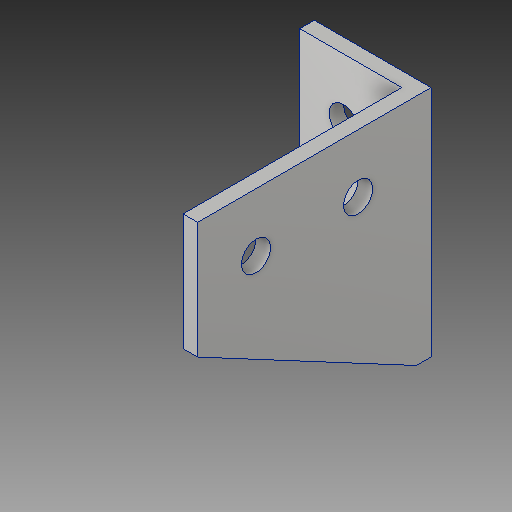
# Autodesk Inventor part: 15102898-16-P-0207
Saved by Autodesk Inventor 2017 (Build 210142000, 142)
## iProperties
Created: 2016-10-02
Part Number: 15102898-16-P-0207
Material: Aluminum 6061
Document SubType Name: Modeling
Designer: gus
Density: 2.7 g/cm^3
Appearance: Aluminum - Flat
Mass: 25.5302 g
Surface Area: 69.3547 cm^2
Volume: 9.45564 cm^3
Author: gus
Autodesk Inventor part; units mm, degrees
ref_plane "YZ Plane" through (0, 0, 0) normal (1, 0, 0) x (0, 1, 0)
ref_plane "XZ Plane" through (0, 0, 0) normal (0, 1, 0) x (-1, 0, 0)
ref_plane "XY Plane" through (0, 0, 0) normal (0, 0, 1) x (1, 0, 0)
sketch "Sketch1" plane through (0, 0, 0) normal (1, 0, 0) x (0, 1, 0)
  line L0 (-25.4, 0) -> (-50.8, -47.625)
  line L1 (-50.8, -47.625) -> (-50.8, -50.8)
  line L2 (-50.8, -50.8) -> (0, -50.8)
  line L3 (0, -50.8) -> (0, 0)
  line L4 (0, 0) -> (-25.4, 0)
  circle A0 centre (-12.7, -12.7) radius 3.175
  circle A1 centre (-12.7, -34.925) radius 3.175
  dimension "d1" = 3.175
  dimension "d2" = 50.8
  dimension "d3" = 50.8
  dimension "d4" = 25.4
  dimension "d5" = 6.35
  dimension "d6" = 6.35
  dimension "d7" = 15.875
  dimension "d8" = 12.7
  dimension "d9" = 12.7
  dimension "d10" = 12.7
  constraints: 10 end point, 3 perpendicular, 2 centre point, 1 coincident, 1 horizontal
  measures "d1" distance of L0.end L1.end
  measures "d2" distance of L1.end L2.end
  measures "d3" distance of L2.end L3.end
  measures "d4" distance of L3.end L0.start
  measures "d5" diameter of A0
  measures "d6" diameter of A1
  measures "d7" distance from line of L2 A1.centre
  measures "d8" distance from line of L3 A1.centre
  measures "d9" distance from line of L3 A0.centre
  measures "d10" distance from line of L4 A0.centre
extrude "Extrusion1" add sketch "Sketch1" along normal blind 3.175
sketch "Sketch2" plane through (0, 0, 0) normal (-1, 0, 0) x (0, 0, 1)
  line L0 (-50.8, -50.8) -> (-50.8, 0) projected
  line L1 (-50.8, 0) -> (0, 0) projected
  line L2 (-50.8, -50.8) -> (-47.625, -50.8)
  line L3 (-47.625, -50.8) -> (-47.625, 0)
  line L4 (-47.625, 0) -> (-50.8, 0)
  line L5 (-50.8, 0) -> (-50.8, -50.8)
  dimension "d13" = 3.175
  constraints: 8 end point, 2 parallel, 1 horizontal, 1 perpendicular, 1 point on line
  measures "d13" distance of L0.start L2.end
extrude "Extrusion2" add sketch "Sketch2" along normal blind 22.225
sketch "Sketch3" plane through (0, -50.8, -47.625) normal (0, 0, 1) x (1, 0, 0)
  circle A0 centre (-12.7, 12.7) radius 3.175
  circle A1 centre (-12.7, 38.1) radius 3.175
  line L0 (-22.225, 50.8) -> (-22.225, 0) projected
  line L1 (0, 50.8) -> (-22.225, 50.8) projected
  line L2 (0, 0) -> (-22.225, 0) projected
  dimension "d16" = 9.525
  dimension "d17" = 12.7
  dimension "d18" = 9.525
  dimension "d19" = 12.7
  dimension "d20" = 6.35
  constraints: 2 centre point, 1 equal radius
  measures "d16" distance from line of L0 A1.centre
  measures "d17" distance from line of L1 A1.centre
  measures "d18" distance from line of L0 A0.centre
  measures "d19" distance from line of L2 A0.centre
  measures "d20" diameter of A0
extrude "Extrusion3" cut sketch "Sketch3" against normal blind 22.225
body "Solid1"
